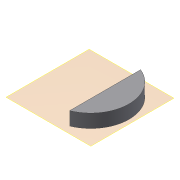
# Autodesk Inventor part: spaceFiller
Saved by Autodesk Inventor 2014 (Build 180170000, 170)
## iProperties
Created: 2016-08-28
Part Number: spaceFiller
Material: Generic
Document SubType Name: Modeling
Designer: Camilo
Density: 1 g/cm^3
Appearance: Default
Author: Camilo
d0: 0.120 mm
d1: 0.120 mm
d2: 5.000 mm
d3: 0.00 deg
Autodesk Inventor part; units mm, degrees
ref_plane "YZ Plane" through (0, 0, 0) normal (1, 0, 0) x (0, 1, 0)
ref_plane "XZ Plane" through (0, 0, 0) normal (0, 1, 0) x (-1, 0, 0)
ref_plane "XY Plane" through (0, 0, 0) normal (0, 0, 1) x (1, 0, 0)
ref_plane "Work Plane1" through (0, 0, 0) normal (0, 0, 1) x (1, 0, 0)
sketch "Sketch1" plane through (0, 0, 0) normal (0, 0, 1) x (1, 0, 0)
  line L0 (5.2722, 6.9481) -> (5.2722, 3.9219) construction
  line L1 (-5.12, 6.9481) -> (-5.12, 3.9219) construction
  arc A0 (-4, 13.8645) -> (4, 13.8645) centre (0, 0) ccw construction
  circle A1 centre (0, 0) radius 14.31
  line L2 (5.3922, 13.2552) -> (5.3922, -13.2552)
  point P0 (0, 0)
  dimension "d0" = 0.12
  dimension "d1" = 0.12
  constraints: 2 end point, 2 point on circle, 1 centre point, 1 coincident
  measures "d0" radial gap between concentric circles of A0 A1
  measures "d1" distance between parallel lines of L0 L2
extrude "Extrusion1" add sketch "Sketch1" along normal blind 5 contours A1 L2 picked at (6.3789, 3.8732)
body "Solid1"
